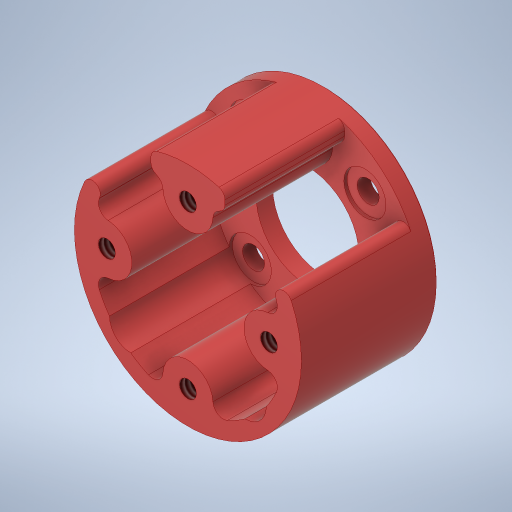
# Autodesk Inventor part: Neo_550_Spacer
Saved by Autodesk Inventor 2023.3 (Build 273359000, 359)
## iProperties
Created: 2024-01-20
Part Number: Neo_550_Spacer
Material: ABS Plastic
Document SubType Name: Modeling
Designer: mavericks
Density: 1.06 g/cm^3
Appearance: Smooth - Red
Author: mavericks
Autodesk Inventor part; units mm, degrees
ref_plane "YZ Plane" through (0, 0, 0) normal (1, 0, 0) x (0, 1, 0)
ref_plane "XZ Plane" through (0, 0, 0) normal (0, 1, 0) x (-1, 0, 0)
ref_plane "XY Plane" through (0, 0, 0) normal (0, 0, 1) x (1, 0, 0)
sketch "Sketch1" plane through (0, 0, 0) normal (0, 0, 1) x (1, 0, 0)
  circle A0 centre (0, 0) radius 17.5
  dimension "d0" = 35
  constraints: 1 centre point, 1 coincident
  measures "d0" diameter of A0
extrude "Extrusion1" add sketch "Sketch1" along normal blind 21
sketch "Sketch2" plane through (0, 0, 21) normal (0, 0, 1) x (1, 0, 0)
  circle A0 centre (0, 0) radius 12.5 construction
  point P0 (0, 12.5)
  point P1 (-12.5, 0)
  point P2 (0, -12.5)
  point P3 (12.5, 0)
  dimension "d3" = 25
  dimension "d6" = 360
  constraints: 2 vertical alignment, 1 coincident, 7 other
hole "Hole1" at (0, 12.5, 21) at (-12.5, 0, 21) at (0, -12.5, 21) at (12.5, 0, 21) direction (0, 0, -1) diameter 2.6416 end through all thread size "6-32 UNC" class "2B" standard "ANSI Unified Screw Threads"
shell "Shell1" thickness 2.54 removed faces 1 at (3.7296, 0.0531, 21)
fillet "Fillet1" radius 1.5875 8 edges at (-14.6058, 3.2359, 11.77) (-14.6058, -3.2359, 11.77) (-3.2359, -14.6058, 11.77) (3.2359, -14.6058, 11.77) (14.6058, -3.2359, 11.77) (14.6058, 3.2359, 11.77) (3.2359, 14.6058, 11.77) (-3.2359, 14.6058, 11.77)
sketch "Sketch3" plane through (0, -12.5, 2.54) normal (0, 0, 1) x (1, 0, 0)
  circle A0 centre (0, 12.5) radius 5.715
  line L0 (-5.715, 12.5) -> (-5.715, 52.9354)
  line L1 (-5.715, 52.9354) -> (5.715, 52.9354)
  line L2 (5.715, 52.9354) -> (5.715, 12.5)
  line L3 (-4.3781, 8.8266) -> (-33.4347, 43.4571)
  line L4 (-33.4347, 43.4571) -> (33.4347, 43.4571)
  line L5 (33.4347, 43.4571) -> (4.3781, 8.8266)
  arc A1 (-12.2985, 8.6445) -> (-12.2985, 16.3555) centre (-12.5, 12.5) ccw projected
  arc A2 (12.2985, 16.3555) -> (12.2985, 8.6445) centre (12.5, 12.5) ccw projected
  point P0 (5.715, 43.4571)
  point P1 (-5.715, 43.4571)
  dimension "d17" = 11.43
  constraints: 12 end point, 5 tangent, 4 point on circle, 2 perpendicular, 1 centre point, 1 coincident, 1 parallel, 1 vertical
  measures "d17" diameter of A0
extrude "Extrusion2" cut sketch "Sketch3" along normal blind 20 contours L2 L4 L5 A0 | A0 L3 L4 L0
fillet "Fillet2" radius 1.27 8 edges at (-15.0097, 8.9977, 11.77) (-13.2645, 6.9177, 11.77) (-5.715, 16.5405, 11.77) (-5.715, 13.7792, 11.7849) (5.715, 16.5405, 11.77) (5.715, 13.7792, 11.7583) (15.0097, 8.9977, 11.77) (13.2645, 6.9177, 11.77)
sketch "Sketch4" plane through (0, 12.5, 2.54) normal (0, 0, 1) x (1, 0, 0)
  circle A0 centre (0, -12.5) radius 7.9375
  dimension "d21" = 15.875
  constraints: 1 centre point, 1 coincident
  measures "d21" diameter of A0
extrude "Extrusion3" cut sketch "Sketch4" against normal through all
chamfer "Chamfer1" distance 0.2 angle 45 1 edges at (-17.5, 0, 0)
sketch "Sketch5" plane through (0, 12.5, 2.54) normal (0, 0, 1) x (1, 0, 0)
  circle A0 centre (0, -12.5) radius 12.5 construction
  circle A1 centre (0, 0) radius 1.3208 construction
  line L0 (-8.8388, -3.6612) -> (0, -12.5) construction
  line L1 (0, -12.5) -> (0, 0) construction
  point P0 (-8.8388, -21.3388)
  point P1 (8.8388, -21.3388)
  point P2 (8.8388, -3.6612)
  dimension "d27" = 45
  dimension "d30" = 360
  constraints: 4 end point, 2 point on circle, 1 centre point, 1 coincident, 1 vertical, 5 other
  measures "d27" angle of L0 L1
hole "Hole2" at (-8.8388, 8.8388, 2.54) at (-8.8388, -8.8388, 2.54) at (8.8388, -8.8388, 2.54) at (8.8388, 8.8388, 2.54) direction (0, 0, -1) diameter 3.4036 end through all start extended yes counterbore diameter 6.5024 counterbore depth 0.5 clearance for "Socket Head Cap Screw" size "M3" standard "Ansi Metric M Profile"
body "Solid1"
